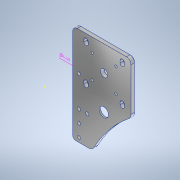
# Autodesk Inventor part: XMotorMount
Saved by Autodesk Inventor 2020 (Build 240168000, 168)
## iProperties
Created: 2018-10-14
Part Number: XMotorMount
Material: Aluminum 6061
Document SubType Name: Modeling
Designer: LillaHunden
Density: 2.7 g/cm^3
Appearance: Aluminum - Flat
Mass: 117.18 g
Surface Area: 185.871 cm^2
Volume: 43.3999 cm^3
Author: LillaHunden
Autodesk Inventor part; units mm, degrees
ref_plane "YZ Plane" through (0, 0, 0) normal (1, 0, 0) x (0, 1, 0)
ref_plane "XZ Plane" through (0, 0, 0) normal (0, 1, 0) x (-1, 0, 0)
ref_plane "XY Plane" through (0, 0, 0) normal (0, 0, 1) x (1, 0, 0)
sketch "Sketch1" plane through (0, 0, 0) normal (0, 0, 1) x (1, 0, 0)
  line L0 (112.0815, -40.6698) -> (40.0716, -40.6698)
  line L1 (40.0716, -40.6698) -> (40.0716, 86.9433)
  line L2 (40.0716, 86.9433) -> (112.0815, 86.9433)
  line L3 (112.0815, 86.9433) -> (112.0815, -40.6698)
  line L4 (40.0716, -40.6698) -> (50.0716, -40.6698) construction
  point P0 (0, 0)
  constraints: 8 end point, 2 parallel, 1 horizontal, 1 perpendicular
extrude "Extrusion1" add sketch "Sketch1" along normal blind 5.15
sketch "Sketch2" plane through (0, 0, 5.15) normal (0, 0, 1) x (1, 0, 0)
  point P0 (0, 0)
sketch "Sketch4" plane through (0, 0, 5.15) normal (0, 0, 1) x (1, 0, 0)
  circle A0 centre (102.6515, 97.6673) radius 2.8 construction
  circle A1 centre (53.4593, 78.9433) radius 2.8 construction
  circle A2 centre (55.5115, 50.5273) radius 2.8 construction
  circle A3 centre (102.6515, 50.5273) radius 2.8 construction
  line L0 (53.4593, 78.9433) -> (53.4593, 75.9433) construction
  line L1 (50.6593, 78.9433) -> (50.6593, 75.9433)
  line L2 (56.2593, 75.9433) -> (56.2593, 78.9433)
  arc A4 (56.2593, 78.9433) -> (50.6593, 78.9433) centre (53.4593, 78.9433) ccw
  arc A5 (50.6593, 75.9433) -> (56.2593, 75.9433) centre (53.4593, 75.9433) ccw
  line L3 (40.0716, 86.9433) -> (40.0716, -40.6698) projected
  line L4 (112.0815, 86.9433) -> (40.0716, 86.9433) projected
  circle A6 centre (53.4593, 77.3133) radius 5 projected
  line L5 (53.4593, 77.3133) -> (53.4593, 77.5733) construction
  point P0 (0, 0)
  point P1 (53.4593, 77.4433)
  point P2 (40.0716, -42.6698)
  point P3 (53.4593, 77.4433)
  dimension "d7" = 3
  dimension "d27" = 5.6
  dimension "d29" = 8
  constraints: 10 end point, 6 centre point, 4 point on circle, 4 tangent, 2 midpoint, 2 parallel, 1 coincident, 1 vertical
  measures "d7" distance of L0.start L0.end
  measures "d27" distance between parallel lines of L1 L2
  measures "d29" distance from line of L4 L0.start
extrude "Extrusion3" cut sketch "Sketch4" against normal through all contours A4 L2 A5 L1
pattern_linear "Rectangular Pattern1" count 2 spacing 47.14 along (1, 0, 0) count 2 spacing 47.14 along (0, -1, 0) of "Extrusion3"
sketch "Sketch9" plane through (0, 0, 5.15) normal (0, 0, 1) x (1, 0, 0)
  point P0 (55.0716, -3.0051)
  point P1 (44.0716, -3.0051)
  point P2 (44.0716, -19.0051)
  point P3 (44.0716, -35.0051)
  point P4 (44.0716, 36.9949)
hole "Hole1" at (55.0716, -3.0051, 5.15) at (44.0716, -3.0051, 5.15) at (44.0716, -19.0051, 5.15) at (44.0716, -35.0051, 5.15) at (44.0716, 36.9949, 5.15) direction (0, 0, -1) diameter 4.4 depth 5.15
sketch "Sketch12" plane through (0, 0, 5.15) normal (0, 0, 1) x (1, 0, 0)
  line L0 (40.0716, -40.6698) -> (112.0815, -40.6698) projected
  arc A0 (112.0815, 21.0326) -> (61.7828, -40.6698) centre (221.9091, -119.8494) ccw
  line L1 (112.0815, -40.6698) -> (112.0815, 86.9433) projected
  point P0 (0, 0)
  constraints: 2 point on circle, 2 point on line, 1 centre point
extrude "Extrusion9" cut sketch "Sketch12" against normal through all
fillet "Fillet1" radius 8 2 edges at (61.7828, -40.6698, 2.575) (112.0815, 21.0326, 2.575)
ref_plane "Work Plane1" through (16.3274, 9.3302, 5.6189) normal (-0.0349258, 0, -0.9993899) x (0, 1, 0)
sketch "Sketch14" plane through (40.0716, -40.6698, 0) normal (-1, 0, 0) x (0, 0, 1)
  line L0 (0, 0) -> (0, 127.6131) projected
  line L1 (0, 0) -> (5.15, 0) projected
  line L2 (5.15, 127.6131) -> (5.15, 0) projected
  line L3 (0, 127.6131) -> (5.15, 127.6131) projected
  point P0 (0, 40.6698)
extrude "Extrusion11" add sketch "Sketch14" along normal blind 4
fillet "Fillet4" radius 4 1 edges at (36.0716, -40.6698, 2.575)
fillet "Fillet5" radius 6 2 edges at (36.0716, 86.9433, 2.575) (112.0815, 86.9433, 2.575)
sketch "Sketch15" plane through (0, 0, 0) normal (0, 0, -1) x (-1, 0, 0)
  circle A0 centre (-77.0293, 53.7433) radius 3.175 construction
  circle A1 centre (-77.0293, 53.7433) radius 3.175 construction
  circle A2 centre (-77.0293, 53.7433) radius 3.475 construction
  circle A3 centre (-77.0293, 53.7433) radius 3.475 construction
  circle A4 centre (-77.0293, 53.7433) radius 4.765
  point P0 (0, 0)
  dimension "d67" = 9.53
  constraints: 1 centre point, 1 coincident
  measures "d67" diameter of A4
extrude "Extrusion12" cut sketch "Sketch15" against normal through all
sketch "Sketch16" plane through (0, 0, 5.15) normal (0, 0, 1) x (1, 0, 0)
  circle A0 centre (76.6012, 9.7443) radius 6.1
  point P0 (0, 0)
  dimension "d68" = 12.2
  constraints: 1 centre point
  measures "d68" diameter of A0
extrude "Extrusion13" cut sketch "Sketch16" against normal through all
sketch "Sketch17" plane through (0, 0, 0) normal (0, 0, -1) x (-1, 0, 0)
  circle A0 centre (-76.7219, 9.782) radius 12.5
  point P0 (0, 0)
  dimension "d71" = 25
  constraints: 1 centre point
  measures "d71" diameter of A0
extrude "Extrusion14" cut sketch "Sketch17" against normal blind 2.75
sketch "Sketch18" plane through (0, 0, 0) normal (0, 0, -1) x (-1, 0, 0)
  circle A0 centre (-92.5293, 69.2433) radius 1.25 construction
  circle A1 centre (-61.5293, 69.2433) radius 1.25 construction
  circle A2 centre (-92.5293, 38.2433) radius 1.25 construction
  circle A3 centre (-61.5293, 38.2433) radius 1.25 construction
  point P0 (0, 0)
hole "Hole2" at (92.5293, 69.2433, 0) at (61.5293, 69.2433, 0) at (61.5293, 38.2433, 0) at (92.5293, 38.2433, 0) direction (0, 0, 1) diameter 3.3 depth 6
chamfer "Chamfer1" distance 0.5 angle 45 28 edges at (81.7943, 53.7433, 0) (89.2219, 9.782, 0) (70.5012, 9.7443, 2.75) (100.5993, 26.0033, 0) (103.3993, 30.3033, 0) (100.5993, 34.6033, 0) (97.7993, 30.3033, 0) (92.5293, 36.5933, 0) (61.5293, 36.5933, 0) (53.4593, 26.0033, 0) (56.2593, 30.3033, 0) (53.4593, 34.6033, 0) (50.6593, 30.3033, 0) (44.0716, 39.1949, 0) (55.0716, -0.8051, 0) (44.0716, -0.8051, 0) (44.0716, -16.8051, 0) (44.0716, -32.8051, 0) (61.5293, 67.5933, 0) (92.5293, 67.5933, 0) (100.5993, 73.1433, 0) (103.3993, 77.4433, 0) (100.5993, 81.7433, 0) (97.7993, 77.4433, 0) (53.4593, 73.1433, 0) (56.2593, 77.4433, 0) (53.4593, 81.7433, 0) (50.6593, 77.4433, 0)
chamfer "Chamfer2" distance 0.5 angle 45 10 edges at (83.7732, -6.5873, 0) (61.0183, -39.5216, 0) (48.4802, -40.6698, 0) (37.2432, -39.4982, 0) (36.0716, 22.1368, 0) (37.829, 85.186, 0) (74.0766, 86.9433, 0) (110.3242, 85.186, 0) (112.0815, 52.9152, 0) (111.3067, 21.4523, 0)
body "Solid1"
